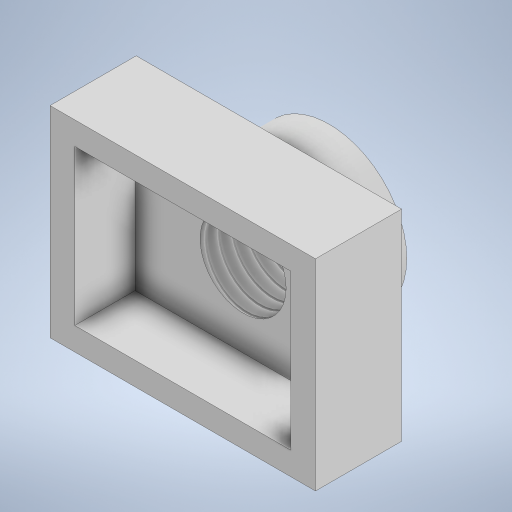
# Autodesk Inventor part: Newairtempguy
Saved by Autodesk Inventor 2023 (Build 270158000, 158)
## iProperties
Created: 2023-02-08
Part Number: Newairtempguy
Material: Generic
Document SubType Name: Modeling
Designer: efarq
Density: 1 g/cm^3
Appearance: Default
Author: efarq
Autodesk Inventor part; units mm, degrees
ref_plane "YZ Plane" through (0, 0, 0) normal (1, 0, 0) x (0, 1, 0)
ref_plane "XZ Plane" through (0, 0, 0) normal (0, 1, 0) x (-1, 0, 0)
ref_plane "XY Plane" through (0, 0, 0) normal (0, 0, 1) x (1, 0, 0)
sketch "Sketch1" plane through (0, 0, 0) normal (0, 0, 1) x (1, 0, 0)
  circle A0 centre (0, 0) radius 5
  circle A1 centre (0, 0) radius 9
  dimension "d0" = 10
  dimension "d1" = 18
  constraints: 2 centre point, 2 coincident
  measures "d0" diameter of A0
  measures "d1" diameter of A1
extrude "Extrusion1" add sketch "Sketch1" along normal blind 7
thread "Thread1" size "M10x1.5" class "6H" standard "ANSI Metric M Profile" full length
sketch "Sketch13" plane through (0, 0, 7) normal (0, 0, 1) x (1, 0, 0)
  line L0 (-15.4051, -11.6713) -> (15.4051, -11.6713)
  line L1 (15.4051, -11.6713) -> (15.4051, 11.6713)
  line L2 (15.4051, 11.6713) -> (-15.4051, 11.6713)
  line L3 (-15.4051, 11.6713) -> (-15.4051, -11.6713)
  line L4 (-15.4051, -11.6713) -> (15.4051, 11.6713) construction
  line L5 (15.4051, -11.6713) -> (-15.4051, 11.6713) construction
  point P0 (0, 0)
  dimension "d50" = 30.8102
  dimension "d51" = 23.3426
  constraints: 12 end point, 2 midpoint, 2 parallel, 1 horizontal, 1 perpendicular
  measures "d50" distance of L2.end L1.end
  measures "d51" distance of L0.end L1.end
extrude "Extrusion13" add sketch "Sketch13" along normal blind 10
sketch "Sketch14" plane through (0, 0, 17) normal (0, 0, 1) x (1, 0, 0)
  line L0 (-12.5334, -9) -> (12.5334, -9)
  line L1 (12.5334, -9) -> (12.5334, 9)
  line L2 (12.5334, 9) -> (-12.5334, 9)
  line L3 (-12.5334, 9) -> (-12.5334, -9)
  line L4 (-12.5334, -9) -> (12.5334, 9) construction
  line L5 (12.5334, -9) -> (-12.5334, 9) construction
  point P0 (0, 0)
  constraints: 12 end point, 2 midpoint, 2 parallel, 1 horizontal, 1 perpendicular
extrude "Extrusion14" cut sketch "Sketch14" against normal blind 7
sketch "Sketch15" plane through (0, 0, 7) normal (0, 0, -1) x (-1, 0, 0)
  circle A0 centre (0, 0) radius 5
  constraints: 1 centre point, 1 coincident
extrude "Extrusion15" cut sketch "Sketch15" against normal blind 7
body "Solid1"
